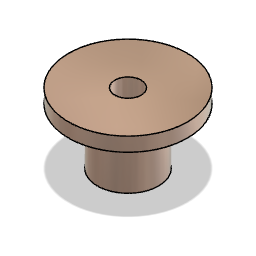
thernal bridge coldhead stage 2 v2 (Autodesk Fusion 360 design; units mm, degrees)
Autodesk Fusion 360 part; units mm, degrees
sketch "Sketch1" plane through (0, 0, 0) normal (0, 0, 1) x (1, 0, 0)
  line L0 (0, 0) -> (34, 0)
  line L1 (34, 0) -> (34, -8)
  line L2 (34, -8) -> (17.5, -8)
  line L3 (17.5, -8) -> (17.5, -40)
  line L4 (17.5, -40) -> (0, -40)
  line L5 (0, -40) -> (0, 0)
  line L6 (7.5, -40) -> (7.5, 0)
  dimension "d1" = 34
  dimension "d2" = 7.5
  dimension "d3" = 10
  dimension "d4" = 8
  dimension "d5" = 40
  constraint coincident L0.start L5.end
  constraint horizontal L0
  constraint perpendicular L0 L1
  constraint perpendicular L1 L2
  constraint perpendicular L2 L3
  constraint perpendicular L3 L4
  constraint perpendicular L0 L5
  constraint coincident L4 L6.start
  constraint coincident L0 L6.end
  constraint perpendicular L0 L6
  measures "d1" distance of L0.start L0.end
  measures "d2" distance of L5 L6
  measures "d3" distance of L3 L6
  measures "d4" distance of L0.end L1.end
  measures "d5" distance of L4.end L0.start
revolve "Revolve1" add sketch "Sketch1" angle 360 about axis through (0, -40, 0) along (0, 1, 0) contours L0 L1 L2 L3 L4 L6
